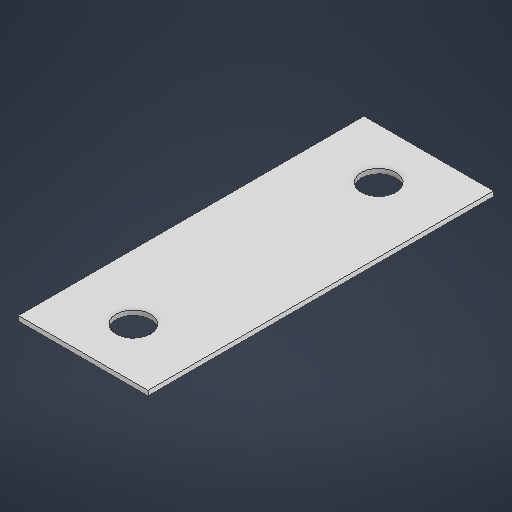
# Autodesk Inventor part: Part18.iptMotorProtector2
Saved by Autodesk Inventor 2026.1 (Build 301233000, 233)
## iProperties
Created: 2026-07-04
Part Number: Part18.iptMotorProtector2
Material: Generic
Document SubType Name: Modeling
Designer: Kasi Pusuluri
Density: 1 g/cm^3
Appearance: Default
Author: Kasi Pusuluri
Autodesk Inventor part; units mm, degrees
ref_plane "YZ Plane" through (0, 0, 0) normal (1, 0, 0) x (0, 1, 0)
ref_plane "XZ Plane" through (0, 0, 0) normal (0, 1, 0) x (-1, 0, 0)
ref_plane "XY Plane" through (0, 0, 0) normal (0, 0, 1) x (1, 0, 0)
sketch "Sketch1" plane through (0, 0, 0) normal (0, 1, 0) x (-1, 0, 0)
  line L0 (0, 0) -> (19.05, 0)
  line L1 (19.05, 0) -> (19.05, -50.8)
  line L2 (19.05, -50.8) -> (0, -50.8)
  line L3 (0, -50.8) -> (0, 0)
  line L4 (19.05, 0) -> (0, 0)
  line L5 (0, 0) -> (0, -14.732)
  line L6 (0, -14.732) -> (19.05, -14.732)
  line L7 (19.05, -14.732) -> (19.05, 0)
  line L8 (19.05, -50.8) -> (0, -50.8)
  line L9 (0, -50.8) -> (0, -36.068)
  line L10 (0, -36.068) -> (19.05, -36.068)
  line L11 (19.05, -36.068) -> (19.05, -50.8)
  circle A0 centre (9.525, -7.366) radius 2.54
  circle A1 centre (9.525, -43.434) radius 2.54
  dimension "d0" = 50.8
  dimension "d1" = 19.05
  dimension "d2" = 14.732
  dimension "d3" = 14.732
  dimension "d4" = 5.08
  dimension "d5" = 5.08
  constraints: 24 end point, 6 parallel, 3 horizontal, 3 perpendicular, 2 centre point, 2 point on line
  measures "d0" distance of L0.end L1.end
  measures "d1" distance of L1.end L2.end
  measures "d2" distance between parallel lines of L6 L0
  measures "d3" distance between parallel lines of L2 L10
  measures "d4" diameter of A0
  measures "d5" diameter of A1
extrude "Extrusion1" add sketch "Sketch1" along normal blind 0.7
equation "\"d3\" = d2"
body "Solid1"
